dehumid_adapter (Autodesk Fusion 360 design; units mm, degrees)
Autodesk Fusion 360 part; units mm, degrees
sketch "Sketch1" plane through (0, 0, 0) normal (0, 1, 0) x (1, 0, 0)
  circle A0 centre (0, 0) radius 13.5
  circle A1 centre (0, 0) radius 16
  line L0 (0, 0) -> (0, -13.5)
  line L1 (0, 0) -> (0, 13.5)
  circle A2 centre (0, 0) radius 30
  dimension "d1" = 2.5
  dimension "d2" = 27
  dimension "d27" = 60
  constraint coincident A0.centre A1.centre
  constraint concentric A0 A1
  constraint coincident A0 L0.end
  constraint vertical L0
  constraint coincident A0 L1.end
  constraint parallel L0 L1
  constraint concentric A0 A2
  measures "d1" distance of A0 A1
  measures "d2" diameter of A0
  measures "d27" diameter of A2
extrude "Extrude1" add sketch "Sketch1" along normal blind 10 and the other way blind 12 contours A1 makes body 1
ref_plane "WorkPlane1" through (0, 0, -20) normal (0, 0, 1) x (1, 0, 0)
sketch "Sketch3" plane through (0, 0, -20) normal (0, 0, 1) x (1, 0, 0)
  circle A0 centre (0, -4.5) radius 5.5
  circle A1 centre (0, -4.5) radius 4.5
  line L0 (0, 0) -> (0, -4.5)
  line L1 (0, -4.5) -> (0, -9)
  dimension "d6" = 9
  dimension "d7" = 11
  constraint concentric A0 A1
  constraint coincident L0.start origin
  constraint vertical L0
  constraint coincident A0.centre A1.centre
  constraint coincident A1 L0.start
  constraint coincident A1 L1.end
  constraint parallel L0 L1
  measures "d6" diameter of A1
  measures "d7" diameter of A0
extrude "Extrude2" add sketch "Sketch3" along normal blind -10 and the other way blind -9 bodies 1
extrude "Extrude3" cut sketch "Sketch1" along normal mid plane 44 contours A0 L0 L1 | A0 L0 L1 bodies 1
extrude "Extrude4" cut sketch "Sketch3" along normal blind 10 contours A1 L0 L1 | A1 L0 L1 bodies 1
sketch "Sketch7" plane through (0, -12, 0) normal (0, -1, 0) x (1, 0, 0)
  circle A0 centre (0, 0) radius 13.5
  circle A1 centre (0, 0) radius 16
  circle A2 centre (0, 0) radius 16
  constraint coincident A0.centre A1.centre
extrude "Extrude5" add sketch "Sketch7" against normal up to surface (3 mm away) contours A0 bodies 1
sketch "Sketch8" plane through (0, 0, 0) normal (1, 0, 0) x (0, 1, 0)
  line L0 (-9, -20) -> (-9, -10)
  line L1 (0, 11) -> (-9, -10)
  line L2 (0, 0) -> (0, 13.5)
  line L3 (0, 11) -> (0, 16)
  line L4 (0, 16) -> (-9, 16)
  line L5 (-9, 16) -> (-9, -10)
  point P0 (-9, -20)
  dimension "d23" = 10
  dimension "d24" = 11
  constraint vertical L0
  constraint coincident P0 L0.start
  constraint coincident L1.start L2
  constraint parallel L2 L3
  constraint perpendicular L3 L4
  constraint perpendicular L4 L5
  constraint coincident L0.end L1.end
  measures "d23" distance of P0 L0.end
  measures "d24" distance of L1.start L2.start
extrude "Extrude6" add sketch "Sketch8" along normal mid plane 34 separate body makes body 2
extrude "Extrude7" cut sketch "Sketch1" against normal blind 25 contours A2 bodies 2
combine "Combine1" operation add target body 2 tool bodies 1
sketch "Sketch9" plane through (0, 0, 0) normal (1, 0, 0) x (0, 1, 0)
  line L0 (-2, 17) -> (-14, -11)
  line L1 (-14, -11) -> (-14, 17)
  line L2 (-14, 17) -> (-2, 17)
  line L3 (0, 11) -> (-9, -10)
  dimension "d31" = 28
  dimension "d32" = 11
  dimension "d33" = 14
  constraint vertical L1
  constraint perpendicular L1 L2
  constraint parallel L0 L3
  measures "d31" distance of L0.end L1.end
  measures "d32" vertical distance of L0.end origin
  measures "d33" horizontal distance of L0.end origin
extrude "Extrude8" [suppressed]
sketch "Sketch5" plane through (0, 0, 0) normal (1, 0, 0) x (0, 1, 0)
  spline S0 degree 5 poles (0, 16) (-1.0827, 15.4586) (-3.0558, 14.1656) (-5.4391, 11.5953) (-7.6175, 7.0378) (-9.1926, -0.2183) (-9.8315, -7.2375) (-10.0328, -13.297) (-10.0437, -17.7278) (-10.0183, -20.0411) knots 0 0 0 0 0 0 0.2 0.4 0.6 0.8 1 1 1 1 1 1
  line L0 (-10.0719, -15.1602) -> (-9.9648, -24.9221)
  line L1 (2, 17) -> (-2, 15)
  line L2 (0, -20) -> (0, -13.5)
  line L3 (1, -20) -> (0, -16)
  spline S1 degree 5 poles (0, 0) (-0.5452, 0) (-1.529, -0.2335) (-2.6852, -1.2835) (-3.6761, -3.8902) (-4.3036, -8.4871) (-4.5057, -12.8216) (-4.5441, -16.3206) (-4.5225, -18.7563) (-4.5, -20) knots 0 0 0 0 0 0 0.2 0.4 0.6 0.8 1 1 1 1 1 1
  line L4 (1, 0) -> (-1, 0)
  point P0 (-4.5, -20)
  constraint midpoint S0.end L0
  constraint midpoint S0.start L1
  constraint vertical L2
  constraint coincident L2 L3.end
  constraint coincident S1.start origin
  constraint coincident P0 S1.end
  constraint midpoint S1.start L4
sketch "Sketch6" plane through (0, 0, 0) normal (0, 1, 0) x (1, 0, 0)
  line L0 (0, 0) -> (0, 20)
  dimension "d12" = 20
  constraint coincident L0.start origin
  constraint vertical L0
  measures "d12" distance of L0.end L0.start
loft "Loft2" [suppressed]
loft "Loft3" [suppressed]
